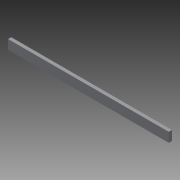
# Autodesk Inventor part: nd-2
Saved by Autodesk Inventor 2015 (Build 190159000, 159)
## iProperties
Created: 2014-07-02
Part Number: nd-2
Material: Generic
Document SubType Name: Modeling
Designer: peter
Density: 1 g/cm^3
Appearance: Default
Author: peter
Autodesk Inventor part; units mm, degrees
ref_plane "YZ Plane" through (0, 0, 0) normal (1, 0, 0) x (0, 1, 0)
ref_plane "XZ Plane" through (0, 0, 0) normal (0, 1, 0) x (-1, 0, 0)
ref_plane "XY Plane" through (0, 0, 0) normal (0, 0, 1) x (1, 0, 0)
sketch "Sketch1" plane through (0, 0, 0) normal (0, 0, 1) x (1, 0, 0)
  line L0 (965.2, 57.2358) -> (0, 57.2358)
  line L1 (965.2, 57.2358) -> (0, 57.2358)
  line L2 (0, 57.2358) -> (0, 0.0858)
  line L3 (0, 0.0858) -> (965.2, 0.0858)
  line L4 (965.2, 0.0858) -> (965.2, 57.2358)
  point P0 (0, 0)
  constraints: 10 end point
extrude "Extrusion1" add sketch "Sketch1" along normal blind 19.05
body "Solid1"
